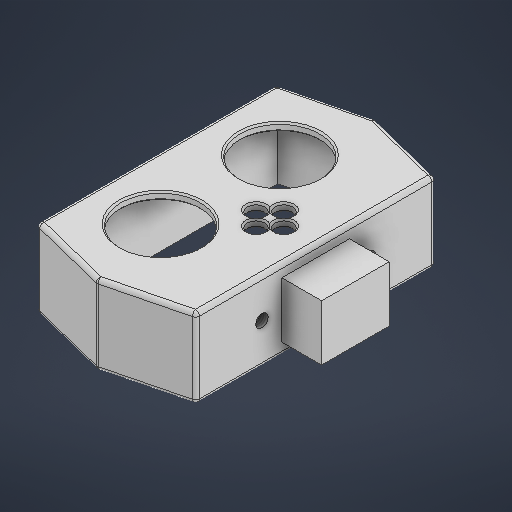
# Autodesk Inventor part: ControllerHousing
Saved by Autodesk Inventor 2026.2 (Build 302298010, 298A)
## iProperties
Created: 2026-02-16
Part Number: ControllerHousing
Material: Generic
Document SubType Name: Modeling
Designer: barbe
Density: 1 g/cm^3
Appearance: Default
Author: barbe
Autodesk Inventor part; units mm, degrees
ref_plane "YZ Plane" through (0, 0, 0) normal (1, 0, 0) x (0, 1, 0)
ref_plane "XZ Plane" through (0, 0, 0) normal (0, 1, 0) x (-1, 0, 0)
ref_plane "XY Plane" through (0, 0, 0) normal (0, 0, 1) x (1, 0, 0)
sketch "Sketch1" plane through (0, 0, 0) normal (0, 1, 0) x (-1, 0, 0)
  line L0 (25.4, 38.1) -> (25.4, -38.1)
  line L1 (-25.4, -38.1) -> (-25.4, 38.1)
  line L2 (-25.4, 38.1) -> (25.4, -38.1) construction
  line L3 (25.4, 38.1) -> (-25.4, -38.1) construction
  line L4 (0, -44.45) -> (25.4, -38.1)
  line L5 (0, -44.45) -> (-25.4, -38.1)
  line L6 (0, 44.45) -> (25.4, 38.1)
  line L7 (0, 44.45) -> (-25.4, 38.1)
  line L8 (25.4, 0) -> (-25.4, 0)
  circle A0 centre (5.08, -19.05) radius 12.7
  circle A1 centre (-6.35, 0) radius 2.794
  circle A2 centre (-15.24, 0) radius 2.794
  line L9 (-10.795, 41.7513) -> (-10.795, -41.7513)
  circle A3 centre (-10.795, -4.445) radius 2.794
  circle A4 centre (5.08, 19.05) radius 12.7
  circle A5 centre (-10.795, 4.445) radius 2.794
  point P0 (0, 0)
  point P1 (-10.795, 0)
  dimension "d0" = 50.8
  dimension "d1" = 76.2
  dimension "d12" = 25.4
  dimension "d19" = 5.588
  constraints: 20 end point, 6 centre point, 5 midpoint, 3 point on line, 2 symmetric about line, 1 parallel, 1 perpendicular, 2 other
  measures "d0" distance of L0.end L1.start
  measures "d1" distance of L0.start L0.end
  measures "d12" diameter of A0
  measures "d19" diameter of A3
extrude "Extrusion3" add sketch "Sketch1" along normal blind 25.4 contours L0 L8 A1 L9 A5 L7 L6 | L0 L4 L5 L9 A3 L8 A1 | L9 A5 L8 A2 L1 L7 | L5 L1 L8 A2 L9 A3
shell "Shell3" thickness 2.54 removed faces 7 at (-22.737, 0, 5.3369) at (-17.7388, 16.9333, -20.0719) at (-17.7388, 16.9333, 18.0281) at (3.5651, 16.9333, -0.2248) at (8.0101, 16.9333, -4.6698) at (12.4551, 16.9333, -0.2248) at (8.0101, 16.9333, 4.2202)
fillet "Fillet3" radius 1.27 18 edges at (-12.7, 25.4, -41.275) (-25.4, 25.4, 0) (-12.7, 25.4, 41.275) (12.7, 25.4, 41.275) (25.4, 25.4, 0) (12.7, 25.4, -41.275) (25.4, 0, 0) (25.4, 12.7, -38.1) (25.4, 12.7, 38.1) (12.7, 0, -41.275) (0, 12.7, -44.45) (-12.7, 0, -41.275) (-25.4, 12.7, -38.1) (-25.4, 0, 0) (-25.4, 12.7, 38.1) (-12.7, 0, 41.275) (0, 12.7, 44.45) (12.7, 0, 41.275)
chamfer "Chamfer1" distance 0.508 angle 45 12 edges at (7.62, 25.4, 19.05) (7.62, 22.86, 19.05) (7.62, 22.86, -19.05) (7.62, 25.4, -19.05) (9.144, 22.86, 0) (13.589, 22.86, 4.445) (18.034, 22.86, 0) (13.589, 22.86, -4.445) (13.589, 25.4, -4.445) (18.034, 25.4, 0) (13.589, 25.4, 4.445) (9.144, 25.4, 0)
sketch "Sketch2" plane through (25.4, 1.27, -37.1084) normal (1, 0, 0) x (0, 0, -1)
  line L0 (-47.9034, 20.319) -> (-26.3134, 20.319)
  line L1 (-26.3134, 20.319) -> (-26.3134, 2.539)
  line L2 (-26.3134, 2.539) -> (-47.9034, 2.539)
  line L3 (-47.9034, 2.539) -> (-47.9034, 20.319)
  line L4 (-47.9034, 20.319) -> (-26.3134, 2.539) construction
  line L5 (-26.3134, 20.319) -> (-47.9034, 2.539) construction
  point P0 (-37.1084, -1.27)
  point P1 (-37.1084, 11.429)
  dimension "d27" = 21.59
  dimension "d28" = 17.78
  constraints: 12 end point, 2 midpoint, 2 parallel, 1 horizontal, 1 perpendicular
  measures "d27" distance of L1.end L2.end
  measures "d28" distance of L0.end L1.end
extrude "Extrusion4" add sketch "Sketch2" along normal blind 12.7
sketch "Sketch3" plane through (25.4, 1.27, -37.1084) normal (1, 0, 0) x (0, 0, -1)
  line L0 (-47.9034, 20.319) -> (-47.9034, 2.539) projected
  point P0 (-37.1084, -1.27)
  point P1 (-54.2534, 11.6635)
  dimension "d31" = 6.35
  measures "d31" distance from line of L0 point (-54.253, 11.664)
hole "Hole1" at (25.4, 12.9335, 17.145) direction (-1, 0, 0) diameter 4 depth 2.54
thread "Thread1" size "M4x0.7" class "6H" standard "ISO Metric profile" full length
mirror "Mirror6" about plane through (0, 0, 0) normal (0, 0, 1) of "Hole1"
thread "Thread2" size "M4x0.7" class "6H" standard "ANSI Metric M Profile" full length
body "Solid3"
